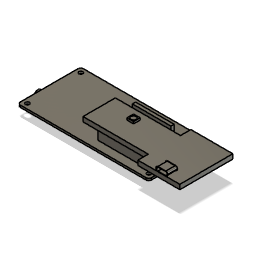
WattWise Open Energy Monitor Casing Version 2 (Autodesk Fusion 360 archive; units mm, degrees)
design "PCB Mockup V2"
Autodesk Fusion 360 part; units mm, degrees
sketch "Sketch1" plane through (0, 0, 0) normal (0, 1, 0) x (1, 0, 0)
  line L0 (47.71, -23.91) -> (-47.71, -23.91)
  line L1 (-49.71, -21.91) -> (-49.71, 21.91)
  line L2 (-47.71, 23.91) -> (47.71, 23.91)
  line L3 (49.71, 21.91) -> (49.71, -21.91)
  line L4 (49.71, -23.91) -> (-49.71, 23.91) construction
  line L5 (-49.71, -23.91) -> (49.71, 23.91) construction
  circle A0 centre (-45.95, 20.28) radius 1.5
  circle A1 centre (46.08, 20.15) radius 1.5
  circle A2 centre (46.08, -20.15) radius 1.5
  circle A3 centre (-46.08, -20.15) radius 1.5
  arc A4 (-47.71, 23.91) -> (-49.71, 21.91) centre (-47.71, 21.91) ccw
  arc A5 (-49.71, -21.91) -> (-47.71, -23.91) centre (-47.71, -21.91) ccw
  arc A6 (47.71, -23.91) -> (49.71, -21.91) centre (47.71, -21.91) ccw
  arc A7 (49.71, 21.91) -> (47.71, 23.91) centre (47.71, 21.91) ccw
  dimension "d1" = 99.42
  dimension "d2" = 47.82
  dimension "d3" = 3
  dimension "d5" = 3.76
  dimension "d6" = 3.63
  dimension "d13" = 3.63
  dimension "d14" = 3.76
  dimension "d15" = 3.76
  dimension "d16" = 3.63
  dimension "d17" = 3.63
  dimension "d18" = 3.76
  dimension "d19" = 2
  constraint horizontal L0
  constraint perpendicular L0 L1
  constraint parallel L0 L2
  constraint parallel L1 L3
  constraint coincident L4 origin
  constraint coincident L5 origin
  constraint equal A2 A3
  constraint equal A0 A3
  constraint equal A0 A1
  constraint coincident L4.end L2
  constraint coincident L4.end L1
  constraint tangent L2 A4
  constraint tangent L1 A4
  constraint coincident L5.start L1
  constraint coincident L5.start L0
  constraint tangent L1 A5
  constraint tangent L0 A5
  constraint equal A4 A5
  constraint coincident L4.start L0
  constraint coincident L4.start L3
  constraint tangent L0 A6
  constraint tangent L3 A6
  constraint equal A4 A6
  constraint coincident L5.end L3
  constraint coincident L5.end L2
  constraint tangent L3 A7
  constraint tangent L2 A7
  constraint equal A4 A7
  measures "d1" distance of L4.end L5.end
  measures "d2" distance of L5.start L4.end
  measures "d3" diameter of A0
  measures "d5" distance of L1 A0.centre
  measures "d6" distance of L2 A0.centre
  measures "d13" distance of L1 A3.centre
  measures "d14" distance of L0 A3.centre
  measures "d15" distance of L0 A2.centre
  measures "d16" distance of L3 A2.centre
  measures "d17" distance of L3 A1.centre
  measures "d18" distance of L2 A1.centre
  measures "d19" radius of A4
extrude "Extrude1" add sketch "Sketch1" along normal blind 1.57 makes body 1
sketch "Sketch2" plane through (0, 1.57, 0) normal (0, 1, 0) x (-1, 0, 0)
  circle A0 centre (45.95, -20.28) radius 1.5
  circle A1 centre (46.08, 20.15) radius 1.5
  circle A2 centre (-46.08, 20.15) radius 1.5
  circle A3 centre (-46.08, -20.15) radius 1.5
  arc A4 (-47.71, 23.91) -> (-49.71, 21.91) centre (-47.71, 21.91) ccw
  line L0 (-49.71, 21.91) -> (-49.71, -21.91)
  arc A5 (-49.71, -21.91) -> (-47.71, -23.91) centre (-47.71, -21.91) ccw
  line L1 (-47.71, -23.91) -> (47.71, -23.91)
  arc A6 (47.71, -23.91) -> (49.71, -21.91) centre (47.71, -21.91) ccw
  line L2 (49.71, -21.91) -> (49.71, 21.91)
  arc A7 (49.71, 21.91) -> (47.71, 23.91) centre (47.71, 21.91) ccw
  line L3 (47.71, 23.91) -> (-47.71, 23.91)
  line L4 (-1.79, -14.04) -> (-31.1, -14.04)
  line L5 (-31.1, -14.04) -> (-31.1, -11.58)
  line L6 (-31.1, -11.58) -> (-1.79, -11.58)
  line L7 (-1.79, -11.58) -> (-1.79, -14.04)
  line L8 (-4.8567, 15.11) -> (-43.63, 15.11)
  line L9 (-43.63, 15.11) -> (-43.63, 17.57)
  line L10 (-43.63, 17.57) -> (-4.8567, 17.57)
  line L11 (-4.8567, 17.57) -> (-4.8567, 15.11)
  line L12 (-4.8567, -4.66) -> (-43.63, -4.66)
  line L13 (-43.63, -4.66) -> (-43.63, -2.2)
  line L14 (-43.63, -2.2) -> (-4.8567, -2.2)
  line L15 (-4.8567, -2.2) -> (-4.8567, -4.66)
  dimension "d23" = 2.46
  dimension "d24" = 29.31
  dimension "d25" = 18.61
  dimension "d28" = 2.46
  dimension "d29" = 2.46
  dimension "d30" = 17.31
  dimension "d31" = 6.34
  dimension "d32" = 6.08
  dimension "d33" = 6.08
  dimension "d34" = 44.8533
  dimension "d52" = 6.92
  constraint horizontal L4
  constraint vertical L5
  constraint horizontal L6
  constraint vertical L7
  constraint horizontal L8
  constraint vertical L9
  constraint horizontal L10
  constraint vertical L11
  constraint horizontal L12
  constraint vertical L13
  constraint horizontal L14
  constraint vertical L15
  constraint equal L8 L12
  measures "d23" distance of L4 L6
  measures "d24" distance of L5 L7
  measures "d25" distance of L0 L5
  measures "d28" distance of L12 L14
  measures "d29" distance of L8 L10
  measures "d30" distance of L8 L14
  measures "d31" distance of L3 L10
  measures "d32" distance of L0 L9
  measures "d33" distance of L0 L13
  measures "d34" distance of L0 L11
  measures "d52" distance of L6 L12
extrude "Extrude2" add sketch "Sketch2" along normal blind 7.79 separate body contours L4 L5 L6 L7 | L8 L9 L10 L11 | L12 L13 L14 L15 makes body 2 at (11.56, 4.1667, -14.04) makes body 3 at (17.7811, 4.1667, -4.66) makes body 4 at (17.7811, 4.1667, 15.11)
sketch "Sketch3" plane through (0, 0, 0) normal (0, -1, 0) x (1, 0, 0)
  circle A0 centre (-45.95, -20.28) radius 1.5
  circle A1 centre (-46.08, 20.15) radius 1.5
  circle A2 centre (46.08, 20.15) radius 1.5
  circle A3 centre (46.08, -20.15) radius 1.5
  arc A4 (49.71, 21.91) -> (47.71, 23.91) centre (47.71, 21.91) ccw
  line L0 (47.71, 23.91) -> (-47.71, 23.91)
  arc A5 (-47.71, 23.91) -> (-49.71, 21.91) centre (-47.71, 21.91) ccw
  line L1 (-49.71, 21.91) -> (-49.71, -21.91)
  arc A6 (-49.71, -21.91) -> (-47.71, -23.91) centre (-47.71, -21.91) ccw
  line L2 (-47.71, -23.91) -> (47.71, -23.91)
  arc A7 (47.71, -23.91) -> (49.71, -21.91) centre (47.71, -21.91) ccw
  line L3 (49.71, -21.91) -> (49.71, 21.91)
  line L4 (-49.71, 10.88) -> (-35.66, 10.88)
  line L5 (-35.66, 10.88) -> (-35.66, -0.67)
  line L6 (-35.66, -0.67) -> (-49.71, -0.67)
  line L7 (-49.71, -0.67) -> (-49.71, 10.88)
  dimension "d37" = 11.55
  dimension "d38" = 14.05
  dimension "d39" = 13.03
  constraint horizontal L4
  constraint vertical L5
  constraint horizontal L6
  constraint vertical L7
  constraint coincident L1 L4.start
  measures "d37" distance of L4 L6
  measures "d38" distance of L5 L7
  measures "d39" distance of L0 L4
extrude "Extrude3" add sketch "Sketch3" along normal blind 6.53 separate body contours L1 L4 L5 L6 L7 makes body 5
sketch "Sketch4" plane through (-49.71, 0, 0) normal (-1, 0, 0) x (0, 0, 1)
  line L0 (10.88, 0) -> (-0.67, 0)
  line L1 (-0.67, 0) -> (-0.67, -6.53)
  line L2 (-0.67, -6.53) -> (10.88, -6.53)
  line L3 (10.88, -6.53) -> (10.88, 0)
  circle A0 centre (5.105, -3.265) radius 2.875
  line L4 (10.88, -3.265) -> (-0.67, -3.265) construction
  dimension "d42" = 5.75
  constraint midpoint L3 L4.start
  constraint midpoint L1 L4.end
  constraint coincident A0.centre L4
  constraint midpoint A0.centre L4
  measures "d42" diameter of A0
extrude "Extrude4" add sketch "Sketch4" along normal blind 3.4 contours A0 bodies 5
sketch "Sketch5" plane through (-53.11, 0, 0) normal (-1, 0, 0) x (0, 0, 1)
  circle A0 centre (5.105, -3.265) radius 2.875
  circle A1 centre (5.105, -3.265) radius 2
  dimension "d45" = 4
  constraint concentric A0 A1
  measures "d45" diameter of A1
extrude "Extrude5" cut sketch "Sketch5" against normal blind 3 contours A1 bodies 5
sketch "Sketch6" plane through (0, 9.36, 0) normal (0, 1, 0) x (-1, 0, 0)
  line L0 (-4.8567, -2.2) -> (-43.63, -2.2)
  line L1 (-43.63, -2.2) -> (-43.63, -4.66)
  line L2 (-43.63, -4.66) -> (-4.8567, -4.66)
  line L3 (-4.8567, -4.66) -> (-4.8567, -2.2)
  line L4 (-44.41, -13.38) -> (-76.2, -13.38)
  line L5 (-76.2, -13.38) -> (-76.2, 26.8)
  line L6 (-76.2, 26.8) -> (-44.41, 26.8)
  line L7 (5.05, 18.96) -> (5.05, -5.54)
  line L8 (-49.71, 21.91) -> (-49.71, -21.91)
  line L9 (-4.8567, 17.57) -> (-43.63, 17.57)
  line L10 (5.05, 18.96) -> (-44.41, 18.96)
  line L11 (5.05, -5.54) -> (-44.41, -5.54)
  line L12 (-44.41, -13.38) -> (-44.41, -5.54)
  line L13 (-44.41, 18.96) -> (-44.41, 26.8)
  dimension "d50" = 26.49
  dimension "d51" = 9.23
  dimension "d53" = 31.79
  dimension "d54" = 24.5
  dimension "d56" = 49.46
  dimension "d57" = 7.84
  dimension "d58" = 7.84
  constraint horizontal L4
  constraint vertical L5
  constraint horizontal L6
  constraint vertical L7
  constraint perpendicular L6 L12
  constraint coincident L10.end L12
  constraint perpendicular L10 L12
  constraint perpendicular L11 L12
  constraint collinear L12 L13
  measures "d50" distance of L5 L8
  measures "d51" distance of L6 L9
  measures "d53" distance of L5 L12
  measures "d54" distance of L10 L11
  measures "d56" distance of L7 L12
  measures "d57" distance of L6 L10
  measures "d58" distance of L4 L11
extrude "Extrude6" add sketch "Sketch6" along normal blind 3.52 separate body contours L0 L1 L2 L3 | L4 L5 L6 L7 L10 L11 L12 L13 makes body 6
sketch "Sketch7" plane through (0, 12.88, 0) normal (0, 1, 0) x (-1, 0, 0)
  line L0 (5.05, 18.96) -> (-44.41, 18.96)
  line L1 (-44.41, 18.96) -> (-44.41, 26.8)
  line L2 (-44.41, 26.8) -> (-76.2, 26.8)
  line L3 (-76.2, 26.8) -> (-76.2, -13.38)
  line L4 (-76.2, -13.38) -> (-44.41, -13.38)
  line L5 (-44.41, -13.38) -> (-44.41, -5.54)
  line L6 (-44.41, -5.54) -> (5.05, -5.54)
  line L7 (5.05, -5.54) -> (5.05, 18.96)
  line L8 (-58.04, 26.8) -> (-67.06, 26.8)
  line L9 (-67.06, 26.8) -> (-67.06, 19.43)
  line L10 (-67.06, 19.43) -> (-58.04, 19.43)
  line L11 (-58.04, 19.43) -> (-58.04, 26.8)
  dimension "d61" = 9.14
  dimension "d62" = 7.37
  dimension "d63" = 9.02
  constraint horizontal L8
  constraint vertical L9
  constraint horizontal L10
  constraint vertical L11
  constraint coincident L2 L8.start
  measures "d61" distance of L3 L9
  measures "d62" distance of L2 L10
  measures "d63" distance of L9 L11
extrude "Extrude7" add sketch "Sketch7" along normal blind 3.44 separate body contours L2 L8 L9 L10 L11 makes body 7
fillet "Fillet1" radius 1.5 4 edges at (58.04, 12.88, 23.115) (58.04, 16.32, 23.115) (67.06, 16.32, 23.115) (67.06, 12.88, 23.115) on bodies 7
shell "Shell1" thickness 0.4 removed faces 1 at (63.5533, 15.1733, 26.8) on bodies 7
sketch "Sketch8" plane through (0, 12.88, 0) normal (0, 1, 0) x (-1, 0, 0)
  line L0 (5.05, 18.96) -> (-44.41, 18.96)
  line L1 (-44.41, 18.96) -> (-44.41, 26.8)
  line L2 (-44.41, 26.8) -> (-76.2, 26.8)
  line L3 (-76.2, 26.8) -> (-76.2, -13.38)
  line L4 (-76.2, -13.38) -> (-44.41, -13.38)
  line L5 (-44.41, -13.38) -> (-44.41, -5.54)
  line L6 (-44.41, -5.54) -> (5.05, -5.54)
  line L7 (5.05, -5.54) -> (5.05, 18.96)
  line L8 (-13.94, -0.36) -> (-18.94, -0.36)
  line L9 (-18.94, -0.36) -> (-18.94, 4.64)
  line L10 (-18.94, 4.64) -> (-13.94, 4.64)
  line L11 (-13.94, 4.64) -> (-13.94, -0.36)
  dimension "d69" = 5
  dimension "d70" = 5
  dimension "d71" = 18.99
  dimension "d72" = 5.18
  constraint horizontal L8
  constraint vertical L9
  constraint horizontal L10
  constraint vertical L11
  measures "d69" distance of L9.end L10.end
  measures "d70" distance of L8 L10
  measures "d71" distance of L7 L11
  measures "d72" distance of L6 L8
extrude "Extrude8" add sketch "Sketch8" along normal blind 1.5 separate body contours L8 L9 L10 L11 makes body 8
sketch "Sketch9" plane through (0, 14.38, 0) normal (0, 1, 0) x (-1, 0, 0)
  line L0 (-13.94, 4.64) -> (-18.94, 4.64)
  line L1 (-18.94, 4.64) -> (-18.94, -0.36)
  line L2 (-18.94, -0.36) -> (-13.94, -0.36)
  line L3 (-13.94, -0.36) -> (-13.94, 4.64)
  circle A0 centre (-16.44, 2.14) radius 1.9979
  line L4 (-16.44, -0.36) -> (-16.44, 4.64) construction
  constraint midpoint L2 L4.start
  constraint midpoint L0 L4.end
  constraint midpoint A0.centre L4
extrude "Extrude9" cut sketch "Sketch9" against normal blind 0.2 contours A0 bodies 8
equation "d13 = PCBhole_shortside"
equation "d14 = PCBhole_longside"
equation "d15 = PCBhole_longside"
equation "d16 = PCBhole_shortside"
equation "d17 = PCBhole_shortside"
equation "d18 = PCBhole_longside"
equation "d20 = PCBthickness"
equation "d23 = HeaderSMD_thickness"
equation "d28 = HeaderSMD_thickness"
equation "d29 = HeaderSMD_thickness"
equation "d35 = HeaderSMD_Height"
equation "d59 = 1.57 mm + 1.95 mm"
equation "PCBthickness = 1.57 mm"
equation "PCBhole_longside = 3.76 mm"
equation "PCBhole_shortside = 3.63 mm"
equation "HeaderSMD_thickness = 2.46 mm"
equation "HeaderSMD_Height = 7.79 mm"

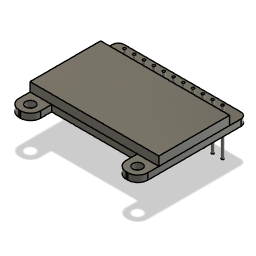
design "TFT Panel"
Autodesk Fusion 360 part; units mm, degrees
sketch "Sketch1" plane through (0, 32, 0) normal (0, 1, 0) x (-1, 0, 0)
  line L0 (47.1, 28.5) -> (-80, 28.5)
  arc A0 (-80, 28.5) -> (-82.5, 26) centre (-80, 26) ccw
  line L1 (-82.5, 26) -> (-82.5, -22)
  arc A1 (-82.5, -22) -> (-80, -24.5) centre (-80, -22) ccw
  line L2 (-80, -24.5) -> (47.1, -24.5)
  arc A2 (47.1, -24.5) -> (49.6, -22) centre (47.1, -22) ccw
  line L3 (49.6, -22) -> (49.6, 26)
  arc A3 (49.6, 26) -> (47.1, 28.5) centre (47.1, 26) ccw
  line L4 (3.205, -6.83) -> (-29.015, -6.83)
  line L5 (-29.015, 10.83) -> (3.205, 10.83)
  line L6 (3.205, 10.83) -> (3.205, -6.83)
  line L7 (-1.185, 10.83) -> (-1.185, -6.83)
  line L8 (-1.985, 10.65) -> (-1.985, -6.65) construction
  line L9 (-29.015, 10.65) -> (-1.985, 10.65) construction
  line L10 (-29.015, -6.65) -> (-29.015, 10.65) construction
  line L11 (-1.985, 2) -> (-29.015, 2) construction
  line L12 (-29.015, -6.65) -> (-29.015, 10.65)
  line L13 (-29.015, 10.65) -> (-1.985, 10.65)
  line L14 (-1.985, 10.65) -> (-1.985, -6.65)
  line L15 (-1.985, -6.65) -> (-29.015, -6.65)
  line L16 (-29.015, -6.65) -> (-29.015, 10.65)
  line L17 (-29.015, 10.65) -> (-1.985, 10.65)
  line L18 (-1.985, 10.65) -> (-1.985, -6.65)
  line L19 (-1.985, -6.65) -> (-29.015, -6.65)
  line L20 (-29.015, 10.65) -> (-1.985, 10.65)
  line L21 (-29.015, 10.83) -> (-29.015, 10.65)
  line L22 (-29.015, -6.83) -> (-29.015, -6.65)
  dimension "d358" = 17.66
  dimension "d359" = 32.22
  constraint horizontal L4
  constraint horizontal L5
  constraint vertical L6
  constraint coincident L5 L7.start
  constraint coincident L4 L7.end
  constraint perpendicular L4 L7
  constraint midpoint L8 L11.start
  constraint midpoint L10 L11.end
  constraint coincident L9.start L10.end
  constraint perpendicular L13 L21
  constraint perpendicular L15 L22
  measures "d358" distance of L4 L5
  measures "d359" distance of L5.start L5.end
extrude "Extrude1" add sketch "Sketch1" against normal blind 2.24 contours L4 L5 L6 L7 | L4 L5 L7 L13 L14 L15 L17 L18 L19 L20 L21 L22 makes body 1
sketch "Sketch2" plane through (0, 29.76, 0) normal (0, -1, 0) x (1, 0, 0)
  line L0 (15.5, -6.45) -> (15.5, 10.45) construction
  line L1 (-1.705, 15.21) -> (27.515, 15.21)
  line L2 (29.015, 13.71) -> (29.015, -9.6)
  line L3 (-3.205, -9.6) -> (-3.205, 13.71)
  line L4 (2.195, -6.83) -> (2.195, -9.6)
  line L5 (23.615, -6.83) -> (23.615, -9.6)
  line L6 (26.515, -12.1) -> (26.115, -12.1)
  line L7 (-0.305, -12.1) -> (-0.705, -12.1)
  arc A0 (26.515, -12.1) -> (29.015, -9.6) centre (26.515, -9.6) ccw
  arc A1 (23.615, -9.6) -> (26.115, -12.1) centre (26.115, -9.6) ccw
  arc A2 (-0.305, -12.1) -> (2.195, -9.6) centre (-0.305, -9.6) ccw
  arc A3 (-3.205, -9.6) -> (-0.705, -12.1) centre (-0.705, -9.6) ccw
  line L8 (26.315, -12.1) -> (26.315, -6.83) construction
  line L9 (-0.505, -12.1) -> (-0.505, -6.83) construction
  circle A4 centre (26.315, -9.465) radius 1.195
  circle A5 centre (-0.505, -9.465) radius 1.195
  arc A6 (-1.705, 15.21) -> (-3.205, 13.71) centre (-1.705, 13.71) ccw
  arc A7 (29.015, 13.71) -> (27.515, 15.21) centre (27.515, 13.71) ccw
  line L10 (29.015, 10.83) -> (-3.205, 10.83)
  line L11 (-3.205, -6.83) -> (29.015, -6.83)
  line L12 (-3.205, 10.83) -> (-3.205, -6.83)
  line L13 (29.015, -6.83) -> (29.015, 10.83)
  line L14 (29.015, -6.83) -> (29.015, -6.65)
  line L15 (29.015, -6.65) -> (1.985, -6.65)
  line L16 (1.985, -6.65) -> (1.985, 10.65)
  line L17 (1.985, 10.65) -> (29.015, 10.65)
  line L18 (29.015, 10.65) -> (29.015, 10.83)
  point P0 (15.5, 2)
  dimension "d241" = 2.5
  dimension "d242" = 2.39
  dimension "d243" = 2.39
  dimension "d244" = 1.5
  dimension "d361" = 5.4
  dimension "d362" = 5.4
  constraint horizontal L1
  constraint perpendicular L1 L2
  constraint parallel L1 L6
  constraint parallel L2 L3
  constraint midpoint L0 P0
  constraint perpendicular L4 L6
  constraint perpendicular L5 L6
  constraint collinear L6 L7
  constraint tangent L2 A0
  constraint tangent L6 A0
  constraint tangent L5 A1
  constraint tangent L6 A1
  constraint equal A0 A1
  constraint tangent L4 A2
  constraint tangent L7 A2
  constraint equal A0 A2
  constraint tangent L3 A3
  constraint tangent L7 A3
  constraint equal A0 A3
  constraint midpoint L6 L8.start
  constraint midpoint L7 L9.start
  constraint midpoint L8 A4.centre
  constraint midpoint L9 A5.centre
  constraint tangent L1 A6
  constraint tangent L3 A6
  constraint tangent L1 A7
  constraint tangent L2 A7
  constraint equal A6 A7
  constraint coincident L4.start L11
  constraint coincident L5.start L11
  constraint collinear L3 L12
  constraint collinear L2 L13
  constraint perpendicular L8 L11
  constraint coincident L8.end L11
  constraint coincident L9.end L11
  constraint perpendicular L9 L11
  measures "d241" radius of A0
  measures "d242" diameter of A4
  measures "d243" diameter of A5
  measures "d244" radius of A6
  measures "d361" distance of L3 L4
  measures "d362" distance of L2 L5
extrude "Extrude2" add sketch "Sketch2" along normal blind 1.6 separate body makes body 2
sketch "Sketch3" plane through (0, 28.16, 0) normal (0, -1, 0) x (1, 0, 0)
  line L0 (-3.205, 13.71) -> (-3.205, -9.6)
  arc A0 (-3.205, -9.6) -> (-0.705, -12.1) centre (-0.705, -9.6) ccw
  line L1 (-0.705, -12.1) -> (-0.305, -12.1)
  arc A1 (-0.305, -12.1) -> (2.195, -9.6) centre (-0.305, -9.6) ccw
  line L2 (2.195, -9.6) -> (2.195, -6.83)
  line L3 (-0.865, 14.12) -> (26.705, 14.12)
  line L4 (26.705, 14.12) -> (26.705, 11.62)
  line L5 (26.705, 11.62) -> (-0.865, 11.62)
  line L6 (-0.865, 14.12) -> (-0.865, 11.62)
  circle A2 centre (26.315, -9.465) radius 1.195
  line L7 (29.015, -9.6) -> (29.015, 13.71)
  arc A3 (29.015, 13.71) -> (27.515, 15.21) centre (27.515, 13.71) ccw
  line L8 (27.515, 15.21) -> (-1.705, 15.21)
  arc A4 (-1.705, 15.21) -> (-3.205, 13.71) centre (-1.705, 13.71) ccw
  line L9 (23.615, -6.83) -> (23.615, -9.6)
  arc A5 (23.615, -9.6) -> (26.115, -12.1) centre (26.115, -9.6) ccw
  line L10 (26.115, -12.1) -> (26.515, -12.1)
  arc A6 (26.515, -12.1) -> (29.015, -9.6) centre (26.515, -9.6) ccw
  line L11 (2.195, -6.83) -> (23.615, -6.83)
  circle A7 centre (-0.505, -9.465) radius 1.195
  dimension "d330" = 2.5
  dimension "d331" = 2.34
  dimension "d367" = 2.31
  constraint perpendicular L5 L6
  measures "d330" distance of L3 L5
  measures "d331" distance of L0 L6
  measures "d367" distance of L4 L7
extrude "Extrude3" add sketch "Sketch3" along normal blind 2 contours L3 L4 L5 L6 bodies 2
sketch "Sketch4" plane through (0, 26.16, 0) normal (0, -1, 0) x (1, 0, 0)
  line L0 (26.705, 14.12) -> (-0.865, 14.12)
  line L1 (-0.865, 14.12) -> (-0.865, 11.62)
  line L2 (-0.865, 11.62) -> (26.705, 11.62)
  line L3 (26.705, 11.62) -> (26.705, 14.12)
  circle A0 centre (3.0507, 12.87) radius 0.325
  circle A1 centre (5.5007, 12.87) radius 0.325
  circle A2 centre (7.9507, 12.87) radius 0.325
  circle A3 centre (10.4007, 12.87) radius 0.325
  circle A4 centre (12.8507, 12.87) radius 0.325
  circle A5 centre (15.3007, 12.87) radius 0.325
  circle A6 centre (17.7507, 12.87) radius 0.325
  circle A7 centre (20.2007, 12.87) radius 0.325
  circle A8 centre (22.6507, 12.87) radius 0.325
  circle A9 centre (25.1007, 12.87) radius 0.325
  circle A10 centre (27.5507, 12.87) radius 0.325
  circle A11 centre (0.6007, 12.9) radius 0.325
  dimension "d336" = 0.65
  dimension "d339" = 24.5
  dimension "d340" = 0
  dimension "d363" = 0.65
  dimension "d364" = 2.45
  measures "d336" diameter of A0
  measures "d363" diameter of A11
  measures "d364" horizontal distance of A0.centre A11.centre
extrude "Extrude4" add sketch "Sketch4" along normal blind 6.5 and the other way blind 5.1 contours A0 | A1 | A2 | A3 | A4 | A5 | A6 | A7 | A8 | A9 | A11 bodies 2
move_body "Move1" bodies 1 2 to x (-1, 0, 0) y (0, 1, 0) z (0, 0, -1) at (31, 0, 4)
sketch "Sketch6" plane through (0, 28.16, 0) normal (0, -1, 0) x (1, 0, 0)
  line L0 (4.295, -10.12) -> (4.295, -7.62)
  line L1 (4.295, -7.62) -> (31.865, -7.62)
  line L2 (31.865, -7.62) -> (31.865, -10.12)
  line L3 (31.865, -10.12) -> (4.295, -10.12)
  circle A0 centre (31.505, 13.465) radius 1.195
  circle A1 centre (4.685, 13.465) radius 1.195
  arc A2 (4.485, 16.1) -> (1.985, 13.6) centre (4.485, 13.6) ccw
  line L4 (1.985, 13.6) -> (1.985, -9.71)
  arc A3 (1.985, -9.71) -> (3.485, -11.21) centre (3.485, -9.71) ccw
  line L5 (3.485, -11.21) -> (32.705, -11.21)
  arc A4 (32.705, -11.21) -> (34.205, -9.71) centre (32.705, -9.71) ccw
  line L6 (34.205, -9.71) -> (34.205, 13.6)
  arc A5 (34.205, 13.6) -> (31.705, 16.1) centre (31.705, 13.6) ccw
  line L7 (31.705, 16.1) -> (31.305, 16.1)
  arc A6 (31.305, 16.1) -> (28.805, 13.6) centre (31.305, 13.6) ccw
  line L8 (28.805, 13.6) -> (28.805, 10.83)
  line L9 (28.805, 10.83) -> (7.385, 10.83)
  line L10 (7.385, 10.83) -> (7.385, 13.6)
  arc A7 (7.385, 13.6) -> (4.885, 16.1) centre (4.885, 13.6) ccw
  line L11 (4.885, 16.1) -> (4.485, 16.1)
  line L12 (34.205, 1.945) -> (1.985, 1.945) construction
  line L13 (2.855, -5.18) -> (18.205, -5.18)
  line L14 (18.205, -5.18) -> (18.205, 9.07)
  line L15 (18.205, 9.07) -> (2.855, 9.07)
  line L16 (2.855, 9.07) -> (2.855, -5.18)
  dimension "d368" = 14.25
  dimension "d369" = 15.35
  dimension "d371" = 16
  dimension "d372" = 7.125
  constraint midpoint L6 L12.start
  constraint midpoint L4 L12.end
  constraint horizontal L13
  constraint vertical L14
  constraint horizontal L15
  constraint vertical L16
  measures "d368" distance of L13 L15
  measures "d369" distance of L14 L16
  measures "d371" distance of L6 L14
  measures "d372" distance of L12 L13
extrude "Extrude5" add sketch "Sketch6" along normal blind 1.63 contours L13 L14 L15 L16 bodies 2
extrude "Extrude6" add 1 faces at (20.005, 30.5067, -6.65) along direction (0, 0, 1) blind 17.3 separate body on bodies 1 makes body 3
combine "Combine1" operation add target body 1 tool bodies 3
